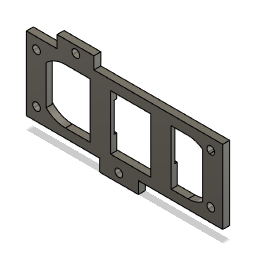
dictofun_1.3_bed_top (Autodesk Fusion 360 design; units mm, degrees)
Autodesk Fusion 360 part; units mm, degrees
sketch "Sketch1" plane through (0, 0, 0) normal (0, 0, 1) x (1, 0, 0)
  circle A0 centre (22.5923, 2.1656) radius 0.95
  arc A1 (9.5633, 18.5906) -> (9.5592, 5.1506) centre (9.5613, 11.8706) ccw
  line L0 (9.5633, 18.5906) -> (39.5595, 18.5815)
  line L1 (39.5253, 5.1415) -> (9.5592, 5.1506)
  circle A2 centre (12.0923, 22.2) radius 0.95
  line L2 (44.5993, 15.8728) -> (44.5993, 7.9997)
  circle A3 centre (2.4923, 18.2) radius 0.95
  circle A4 centre (45.0923, 6.1656) radius 0.95
  circle A5 centre (2.4923, 6.1656) radius 0.95
  circle A6 centre (45.0923, 18.2) radius 0.95
  line L3 (0, 3) -> (3.0006, 3)
  line L4 (0, 3) -> (17.9234, 2.9641)
  line L5 (27.4015, 2.9451) -> (48, 2.9039)
  line L6 (17.9234, 0) -> (27.4015, 0)
  line L7 (48, 20.927) -> (48, 2.9039)
  line L8 (16.5, 20.9269) -> (48, 20.927)
  line L9 (0, 20.927) -> (7.5, 20.927)
  line L10 (7.5, 23.9269) -> (16.5216, 23.9269)
  line L11 (16.5216, 23.9269) -> (16.5, 20.9269)
  line L12 (7.5, 20.927) -> (7.5, 23.9269)
  line L13 (0, 20.927) -> (0, 3)
  line L14 (17.9234, 2.9641) -> (17.9234, 0)
  line L15 (17.9234, 0) -> (27.4015, 0)
  line L16 (27.4015, 0) -> (27.4015, 2.9451)
  arc A7 (44.5993, 15.8728) -> (39.5595, 18.5815) centre (39.5577, 12.5354) ccw
  arc A8 (39.5253, 5.1415) -> (44.5993, 7.9997) centre (39.5271, 11.0712) ccw
  dimension "d15" = 9.6
  dimension "d16" = 4
  dimension "d17" = 4
  dimension "d18" = 12.0344
  dimension "d19" = 42.6
  dimension "d20" = 20.1
  dimension "d21" = 1.9
  dimension "d22" = 1.9
  dimension "d23" = 1.9
  dimension "d24" = 1.9
  dimension "d25" = 1.9
  dimension "d26" = 1.9
  dimension "d29" = 9
  dimension "d31" = 7.5
  dimension "d32" = 3
  constraint collinear L4 L5
  constraint collinear L8 L9
  constraint tangent L1 A8
  constraint tangent A1 L1
  constraint tangent A1 L0
  constraint tangent L0 A7
  constraint vertical L2
  measures "d15" horizontal distance of A2.centre A3.centre
  measures "d16" vertical distance of A2.centre A3.centre
  measures "d17" vertical distance of A0.centre A5.centre
  measures "d18" distance of A3.centre A5.centre
  measures "d19" distance of A3.centre A6.centre
  measures "d20" horizontal distance of A0.centre A5.centre
  measures "d21" diameter of A2
  measures "d22" diameter of A3
  measures "d23" diameter of A5
  measures "d24" diameter of A0
  measures "d25" diameter of A4
  measures "d26" diameter of A6
  measures "d29" distance of L9.end L8.start
  measures "d31" distance of L12 L13
  measures "d32" distance of L8.start L10
extrude "Extrude1" add sketch "Sketch1" along normal blind 0.2
sketch "Sketch4" plane through (0, 0, 0.2) normal (0, 0, 1) x (1, 0, 0)
  circle A0 centre (2.4923, 6.1656) radius 0.95
  circle A1 centre (45.0923, 6.1656) radius 0.95
  arc A2 (9.5633, 18.5906) -> (9.5592, 5.1506) centre (9.5613, 11.8706) ccw
  line L0 (9.5633, 18.5906) -> (39.5595, 18.5815)
  arc A3 (44.5993, 15.8728) -> (39.5595, 18.5815) centre (39.5577, 12.5354) ccw
  line L1 (44.5993, 15.8728) -> (44.5993, 7.9997)
  arc A4 (39.5253, 5.1415) -> (44.5993, 7.9997) centre (39.5271, 11.0712) ccw
  line L2 (39.5253, 5.1415) -> (9.5592, 5.1506)
  circle A5 centre (45.0923, 18.2) radius 0.95
  circle A6 centre (22.5923, 2.1656) radius 0.95
  circle A7 centre (12.0923, 22.2) radius 0.95
  circle A8 centre (2.4923, 18.2) radius 0.95
  line L3 (0, 20.927) -> (0, 3)
  line L4 (0, 3) -> (17.9234, 2.9641)
  line L5 (17.9234, 2.9641) -> (17.9234, 0)
  line L6 (17.9234, 0) -> (27.4015, 0)
  line L7 (27.4015, 0) -> (27.4015, 2.9451)
  line L8 (27.4015, 2.9451) -> (48, 2.9039)
  line L9 (48, 2.9039) -> (48, 20.927)
  line L10 (48, 20.927) -> (16.5, 20.9269)
  line L11 (16.5, 20.9269) -> (16.5216, 23.9269)
  line L12 (16.5216, 23.9269) -> (7.5, 23.9269)
  line L13 (7.5, 23.9269) -> (7.5, 20.927)
  line L14 (7.5, 20.927) -> (0, 20.927)
sketch "Sketch5" plane through (0, 0, 0.2) normal (0, 0, 1) x (1, 0, 0)
  line L0 (0, 20.927) -> (4.8413, 20.927)
  line L1 (4.8413, 20.927) -> (4.8413, 3)
  line L2 (4.8413, 3) -> (0, 3)
  line L3 (0, 3) -> (0, 20.927)
  arc A0 (9.5633, 18.5906) -> (9.5592, 5.1506) centre (9.5613, 11.8706) ccw
  line L4 (48, 20.927) -> (43.0993, 20.927)
  line L5 (43.0993, 20.927) -> (43.0993, 2.927)
  line L6 (43.0993, 2.927) -> (48, 2.927)
  line L7 (48, 2.927) -> (48, 20.927)
  line L8 (44.5993, 15.8728) -> (44.5993, 7.9997)
  line L9 (48, 2.9039) -> (48, 20.927)
  line L10 (15.6, 20.9269) -> (20.6, 20.9269)
  line L11 (20.6, 20.9269) -> (20.6, 3)
  line L12 (20.6, 3) -> (15.6, 3)
  line L13 (15.6, 3) -> (15.6, 20.9269)
  line L14 (35.4, 2.9291) -> (30.4, 2.9391)
  line L15 (30.4, 2.9391) -> (30.4, 20.927)
  line L16 (30.4, 20.927) -> (35.4, 20.927)
  line L17 (35.4, 20.927) -> (35.4, 2.9291)
  circle A1 centre (45.0932, 6.1683) radius 0.9453
  circle A2 centre (45.1, 18.2) radius 0.9525
  line L18 (48, 20.927) -> (16.5, 20.9269)
  line L19 (7.5, 20.927) -> (0, 20.927)
  line L20 (27.4015, 2.9451) -> (48, 2.9039)
  dimension "d33" = 6.72
  dimension "d34" = 4.72
  dimension "d35" = 1.5
  dimension "d37" = 15.6
  dimension "d38" = 5
  dimension "d39" = 17.6
  dimension "d40" = 5
  constraint horizontal L0
  constraint vertical L1
  constraint horizontal L2
  constraint vertical L3
  constraint horizontal L4
  constraint vertical L5
  constraint horizontal L6
  constraint vertical L7
  constraint collinear L7 L9
  constraint horizontal L10
  constraint vertical L11
  constraint horizontal L12
  constraint vertical L13
  constraint vertical L15
  constraint horizontal L16
  constraint vertical L17
  constraint collinear L16 L18
  constraint collinear L10 L18
  constraint collinear L0 L19
  constraint collinear L14 L20
  measures "d33" radius of A0
  measures "d34" distance of L1 A0.centre
  measures "d35" distance of L5 L8
  measures "d37" distance of L3 L13
  measures "d38" distance of L11 L13
  measures "d39" distance of L7 L15
  measures "d40" distance of L15 L17
extrude "Extrude4" add sketch "Sketch4" sketch "Sketch5" along normal blind 1.5 of sketch 2 contours L1 A0 | L4 L5 L6 L7 L9 L18 | L14 L15 L16 L17 L18 L20 | L10 L11 L12 L13 L18
sketch "Sketch7" plane through (0, 0, 0) normal (0, 0, -1) x (-1, 0, 0)
  circle A0 centre (-22.5923, 2.1656) radius 0.95
  circle A1 centre (-2.4923, 6.1656) radius 0.95
  arc A2 (-9.5592, 5.1506) -> (-9.5633, 18.5906) centre (-9.5613, 11.8706) ccw
  line L0 (-9.5592, 5.1506) -> (-39.5253, 5.1415)
  arc A3 (-44.5993, 7.9997) -> (-39.5253, 5.1415) centre (-39.5271, 11.0712) ccw
  line L1 (-44.5993, 7.9997) -> (-44.5993, 15.8728)
  arc A4 (-39.5595, 18.5815) -> (-44.5993, 15.8728) centre (-39.5577, 12.5354) ccw
  line L2 (-39.5595, 18.5815) -> (-9.5633, 18.5906)
  circle A5 centre (-45.0923, 6.1656) radius 0.95
  circle A6 centre (-45.0923, 18.2) radius 0.95
  circle A7 centre (-12.0923, 22.2) radius 0.95
  circle A8 centre (-2.4923, 18.2) radius 0.95
  line L3 (0, 3) -> (0, 20.927)
  line L4 (0, 20.927) -> (-7.5, 20.927)
  line L5 (-7.5, 20.927) -> (-7.5, 23.9269)
  line L6 (-7.5, 23.9269) -> (-16.5216, 23.9269)
  line L7 (-16.5216, 23.9269) -> (-16.5, 20.9269)
  line L8 (-16.5, 20.9269) -> (-48, 20.927)
  line L9 (-48, 20.927) -> (-48, 2.9039)
  line L10 (-48, 2.9039) -> (-27.4015, 2.9451)
  line L11 (-27.4015, 2.9451) -> (-27.4015, 0)
  line L12 (-27.4015, 0) -> (-17.9234, 0)
  line L13 (-17.9234, 0) -> (-17.9234, 2.9641)
  line L14 (-17.9234, 2.9641) -> (0, 3)
  line L15 (-21.2636, 16.1269) -> (-15.1351, 16.1269)
  line L16 (-15.1351, 16.1269) -> (-15.1351, 8.9)
  line L17 (-15.1351, 8.9) -> (-21.2636, 8.9)
  line L18 (-21.2636, 8.9) -> (-21.2636, 16.1269)
  line L19 (-36.0884, 17.5826) -> (-29.6453, 17.5826)
  line L20 (-29.6453, 17.5826) -> (-29.6453, 10.0771)
  line L21 (-29.6453, 10.0771) -> (-36.0884, 10.0771)
  line L22 (-36.0884, 10.0771) -> (-36.0884, 17.5826)
  dimension "d43" = 4.8
  dimension "d44" = 8.9
  dimension "d45" = 1
  constraint horizontal L15
  constraint vertical L16
  constraint horizontal L17
  constraint vertical L18
  constraint horizontal L19
  constraint vertical L20
  constraint horizontal L21
  constraint vertical L22
  measures "d43" distance of L7.end L15
  measures "d44" distance of L12.end L17
  measures "d45" distance of L2 L19.start
extrude "Extrude5" cut sketch "Sketch7" against normal blind 0.8 contours L15 L16 L17 L18 | L19 L20 L21 L22
equation "d22 = d21"
equation "d23 = d21"
equation "d24 = d21"
equation "d25 = d21"
equation "d26 = d21"
equation "d34 = d33 - 2 mm"
